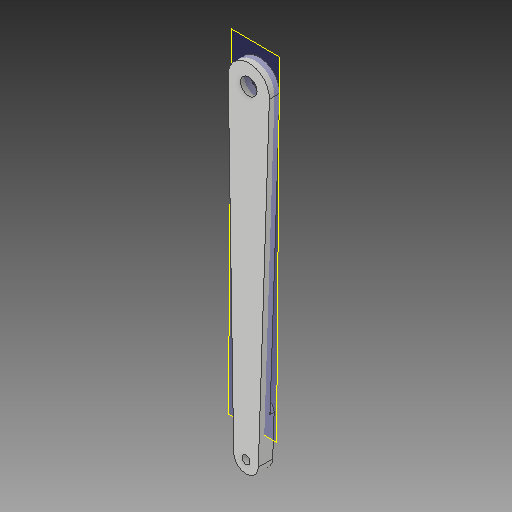
# Autodesk Inventor part: RightArm
Saved by Autodesk Inventor 2018 (Build 220112000, 112)
## iProperties
Created: 2020-03-25
Part Number: RightArm
Material: Generic
Document SubType Name: Modeling
Designer: technik
Density: 1 g/cm^3
Appearance: Default
Author: technik
Autodesk Inventor part; units mm, degrees
ref_plane "YZ Plane" through (0, 0, 0) normal (1, 0, 0) x (0, 1, 0)
ref_plane "XZ Plane" through (0, 0, 0) normal (0, 1, 0) x (-1, 0, 0)
ref_plane "XY Plane" through (0, 0, 0) normal (0, 0, 1) x (1, 0, 0)
sketch "Sketch1" plane through (0, 0, 0) normal (0, 0, 1) x (1, 0, 0)
  circle A0 centre (0, 0) radius 0.5
  spline S0 degree 3 poles (0.2195, 78.8895) (0.2199, 78.9523) (0.2329, 79.0192) (0.2847, 79.142) (0.3236, 79.198) (0.413, 79.2862) (0.4694, 79.3243) (0.5929, 79.3745) (0.66, 79.3866) (0.7856, 79.3858) (0.8524, 79.3728) (0.9753, 79.321) (1.0313, 79.2822) (1.1195, 79.1928) (1.1576, 79.1363) (1.2078, 79.0128) (1.2199, 78.9458) (1.2191, 78.8202) (1.2061, 78.7533) (1.1543, 78.6305) (1.1154, 78.5745) (1.0261, 78.4863) (0.9696, 78.4482) (0.8461, 78.398) (0.779, 78.3858) (0.6535, 78.3867) (0.5866, 78.3996) (0.4637, 78.4515) (0.4078, 78.4903) (0.3196, 78.5797) (0.2815, 78.6362) (0.2312, 78.7597) (0.2191, 78.8267) (0.2195, 78.8895) knots 0 0 0 0 0.0625 0.0625 0.125 0.125 0.1875 0.1875 0.25 0.25 0.3125 0.3125 0.375 0.375 0.4375 0.4375 0.5 0.5 0.5625 0.5625 0.625 0.625 0.6875 0.6875 0.75 0.75 0.8125 0.8125 0.875 0.875 0.9375 0.9375 1 1 1 1
  line L0 (0.6862, 78.8895) -> (0, 0)
  circle A1 centre (0, 0) radius 3
  circle A2 centre (0.6862, 78.8895) radius 5
  line L1 (5.6833, 78.7193) -> (2.9983, -0.1021)
  line L2 (-2.9996, -0.05) -> (-4.3131, 78.8063)
  circle A3 centre (0, 0) radius 0.75
  point P0 (0, 0)
  point P1 (0.2195, 78.8895)
  dimension "d0" = 6
  dimension "d1" = 10
  dimension "d12" = 1.5
  constraints: 6 end point, 4 point on circle, 4 tangent, 3 centre point, 3 coincident
  measures "d0" diameter of A1
  measures "d1" diameter of A2
  measures "d12" diameter of A3
extrude "Extrusion1" add sketch "Sketch1" along normal blind 3.5 contours A2 L1 A1 L0 | L0 A1 L2 A2 | A2 | A1 | A3
sketch "Sketch2" plane through (5.6833, 78.7193, 3.5) normal (0.9994203, -0.0340447, 0) x (0, 0, -1)
  line L0 (3.5, -66.8672) -> (2.5, -66.8672)
  line L1 (2.5, -66.8672) -> (2.5, 7.5211)
  line L2 (2.5, 7.5211) -> (3.5, 7.5211)
  line L3 (3.5, 7.5211) -> (3.5, -66.8672)
  line L4 (3.5, -81.8672) -> (0, -81.8672) projected
  line L5 (3.5, -78.8672) -> (3.5, 0) projected
  dimension "d4" = 1
  dimension "d5" = 15
  constraints: 8 end point, 2 parallel, 1 collinear, 1 horizontal, 1 perpendicular
  measures "d4" distance of L1.end L2.end
  measures "d5" distance between parallel lines of L4 L0
extrude "Extrusion2" cut sketch "Sketch2" against normal through all
fillet "Fillet1" radius 2 2 edges at (3.4068, 11.8909, 0.5) (-3.2022, 12.116, 0.5)
ref_plane "Work Plane1" through (0.6862, 78.8895, 2.25) normal (0, 0, -1) x (-0.9999622, 0.0086975, 0)
sketch "Sketch3" plane through (0.6862, 78.8895, 2.25) normal (0, 0, -1) x (-0.9999622, 0.0086975, 0)
  arc A0 (0, -2.375) -> (0, 2.375) centre (0, 0) ccw
  line L0 (0, 2.375) -> (0, -2.375)
  point P0 (0, -78.8925)
  dimension "d10" = 4.75
  constraints: 2 end point, 2 point on circle, 1 centre point, 1 vertical, 1 other
  measures "d10" diameter of A0
revolve "Revolution1" cut sketch "Sketch3" angle 360 about axis through (0.7068, 81.2645, 2.25) along (-0.0086975, -0.9999622, 0)
sketch "Sketch4" plane through (0, 0, 3.5) normal (0, 0, 1) x (1, 0, 0)
  circle A0 centre (0, 0) radius 0.5 projected
  circle A1 centre (0, 0) radius 1
  point P0 (0, 0)
  dimension "d13" = 2
  constraints: 1 centre point, 1 coincident
  measures "d13" diameter of A1
extrude "Extrusion3" cut sketch "Sketch4" against normal through all
body "Solid1"
